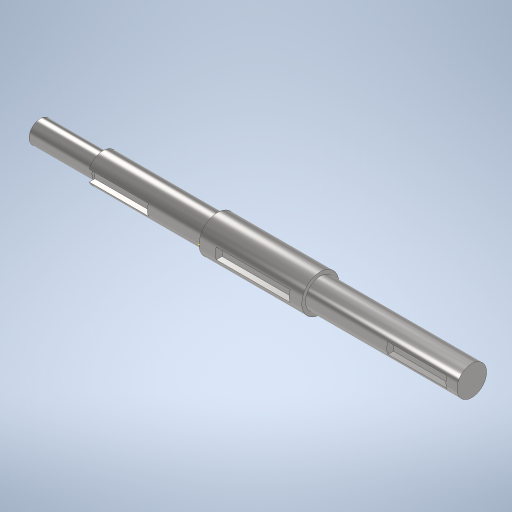
# Autodesk Inventor part: shoulder1_shaft
Saved by Autodesk Inventor 2024 (Build 280153000, 153)
## iProperties
Created: 2025-08-07
Part Number: shoulder1_shaft
Material: 鋼、炭素鋼
Document SubType Name: Modeling
Designer: HosodaLab2
Density: 7.85 g/cm^3
Appearance: 半つや出し
材料: S45C
個数: 1
Author: HosodaLab2
Autodesk Inventor part; units mm, degrees
ref_plane "YZ Plane" through (0, 0, 0) normal (1, 0, 0) x (0, 1, 0)
ref_plane "XZ Plane" through (0, 0, 0) normal (0, 1, 0) x (-1, 0, 0)
sketch "スケッチ1" plane through (0, 0, 0) normal (0, 1, 0) x (-1, 0, 0)
  circle A0 centre (0, 0) radius 5
  dimension "d0" = 10
  constraints: 1 centre point, 1 coincident
  measures "d0" diameter of A0
extrude "押し出し1" add sketch "スケッチ1" along normal blind 27.8
sketch "スケッチ2" plane through (0, 27.8, 0) normal (0, 1, 0) x (1, 0, 0)
  circle A0 centre (0, 0) radius 4
  dimension "d3" = 8
  constraints: 1 centre point, 1 coincident
  measures "d3" diameter of A0
extrude "押し出し2" add sketch "スケッチ2" along normal blind 41
sketch "スケッチ3" plane through (0, 68.8, 0) normal (0, 1, 0) x (1, 0, 0)
  circle A0 centre (0, 0) radius 3
  dimension "d6" = 6
  constraints: 1 centre point, 1 coincident
  measures "d6" diameter of A0
extrude "押し出し3" [suppressed]
sketch "スケッチ4" plane through (0, 0, 0) normal (0, -1, 0) x (1, 0, 0)
  circle A0 centre (0, 0) radius 4 projected
  circle A1 centre (0, 0) radius 4
  dimension "d9" = 8
  constraints: 1 centre point, 1 coincident
  measures "d9" diameter of A1
extrude "押し出し4" add sketch "スケッチ4" along normal blind 31
sketch "スケッチ5" plane through (0, -31, 0) normal (0, -1, 0) x (1, 0, 0)
  circle A0 centre (0, 0) radius 4 projected
  circle A1 centre (0, 0) radius 3
  dimension "d12" = 6
  constraints: 1 centre point, 1 coincident
  measures "d12" diameter of A1
extrude "押し出し5" add sketch "スケッチ5" along normal blind 17 contours A1
sketch "スケッチ6" plane through (0, 0, 0) normal (0, -1, 0) x (1, 0, 0)
  circle A0 centre (0, 0) radius 5 projected
  point P0 (5, 0)
  constraints: 1 horizontal alignment, 1 other
ref_plane "作業平面1" through (5, 0, 0) normal (1, 0, 0) x (0, 1, 0)
sketch "スケッチ7" plane through (5, 0, 0) normal (1, 0, 0) x (0, 1, 0)
  line L0 (4.4, 1.5) -> (24.4, 1.5)
  line L1 (24.4, 1.5) -> (24.4, -1.5)
  line L2 (24.4, -1.5) -> (4.4, -1.5)
  line L3 (4.4, -1.5) -> (4.4, 1.5)
  line L4 (4.4, 1.5) -> (24.4, -1.5) construction
  line L5 (24.4, 1.5) -> (4.4, -1.5) construction
  line L6 (0, -5) -> (0, 5) projected
  point P0 (0, 0)
  point P1 (14.4, 0)
  dimension "d15" = 20
  dimension "d16" = 3
  dimension "d17" = 4.4
  constraints: 12 end point, 2 midpoint, 2 parallel, 1 horizontal, 1 perpendicular
  measures "d15" distance of L1.end L2.end
  measures "d16" distance of L0.end L1.end
  measures "d17" distance between parallel lines of L6 L3
extrude "押し出し6" cut sketch "スケッチ7" against normal blind 1.8
sketch "スケッチ8" plane through (5, 0, 0) normal (1, 0, 0) x (0, 1, 0)
  point P0 (0, 0)
sketch "スケッチ9" plane through (5, 0, 0) normal (1, 0, 0) x (0, 1, 0)
  point P0 (0, 0)
ref_plane "作業平面2" through (4, 0, 0) normal (1, 0, 0) x (0, 1, 0)
sketch "スケッチ10" plane through (4, 0, 0) normal (1, 0, 0) x (0, 1, 0)
  line L0 (49.8, 1.5) -> (65.8, 1.5)
  line L1 (65.8, 1.5) -> (65.8, -1.5)
  line L2 (65.8, -1.5) -> (49.8, -1.5)
  line L3 (49.8, -1.5) -> (49.8, 1.5)
  line L4 (49.8, 1.5) -> (65.8, -1.5) construction
  line L5 (65.8, 1.5) -> (49.8, -1.5) construction
  line L6 (-31, 1.5) -> (-15, 1.5)
  line L7 (-15, 1.5) -> (-15, -1.5)
  line L8 (-15, -1.5) -> (-31, -1.5)
  line L9 (-31, -1.5) -> (-31, 1.5)
  line L10 (-31, 1.5) -> (-15, -1.5) construction
  line L11 (-15, 1.5) -> (-31, -1.5) construction
  line L12 (-31, 4) -> (-31, -4) projected
  line L13 (68.8, -4) -> (68.8, 4) projected
  point P0 (0, 0)
  point P1 (57.8, 0)
  point P2 (-23, 0)
  dimension "d21" = 16
  dimension "d22" = 3
  dimension "d23" = 16
  dimension "d24" = 3
  dimension "d25" = 0
  dimension "d26" = 3
  constraints: 24 end point, 4 midpoint, 4 parallel, 2 horizontal, 2 perpendicular
  measures "d21" distance of L1.end L2.end
  measures "d22" distance of L0.end L1.end
  measures "d23" distance of L7.end L8.end
  measures "d24" distance of L6.end L7.end
  measures "d25" distance between parallel lines of L9 L12
  measures "d26" distance between parallel lines of L13 L1
extrude "押し出し8" cut sketch "スケッチ10" against normal blind 1.8
